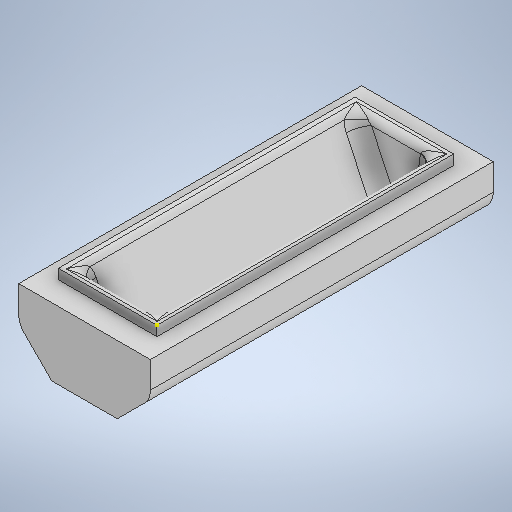
# Autodesk Inventor part: E1-QR-Port
Saved by Autodesk Inventor 2025.2 (Build 292293000, 293)
## iProperties
Created: 2025-11-18
Part Number: E1-QR-Port
Material: 일반
Document SubType Name: Modeling
Designer: RunGeun
Density: 1 g/cm^3
Appearance: 기본값
Author: RunGeun
Autodesk Inventor part; units mm, degrees
ref_plane "YZ Plane" through (0, 0, 0) normal (1, 0, 0) x (0, 1, 0)
ref_plane "XZ Plane" through (0, 0, 0) normal (0, 1, 0) x (-1, 0, 0)
ref_plane "XY Plane" through (0, 0, 0) normal (0, 0, 1) x (1, 0, 0)
sketch "스케치1" plane through (0, 0, 0) normal (0, 1, 0) x (-1, 0, 0)
  line L0 (0, 0) -> (29.8, 0)
  line L1 (29.8, 0) -> (29.8, -89.7)
  line L2 (29.8, -89.7) -> (0, -89.7)
  line L3 (0, -89.7) -> (0, 0)
  line L4 (34.8, 7) -> (-5, 7)
  line L5 (-5, 7) -> (-5, -96.7)
  line L6 (-5, -96.7) -> (34.8, -96.7)
  line L7 (34.8, -96.7) -> (34.8, 7)
  line L8 (16.2, -3) -> (6, -3)
  line L9 (6, -3) -> (6, -86.7)
  line L10 (6, -86.7) -> (16.2, -86.7)
  line L11 (16.2, -86.7) -> (16.2, -3)
  point P0 (11.1, -86.7)
  dimension "d0" = 89.7
  dimension "d1" = 29.8
  dimension "d2" = 7
  dimension "d3" = 5
  dimension "d4" = 7
  dimension "d5" = 5
  dimension "d6" = 3
  dimension "d7" = 3
  dimension "d8" = 13.6
  dimension "d9" = 6
  constraints: 24 end point, 6 parallel, 3 horizontal, 3 perpendicular, 1 midpoint
  measures "d0" distance of L2.end L0.start
  measures "d1" distance of L1.end L2.end
  measures "d2" distance between parallel lines of L6 L2
  measures "d3" distance between parallel lines of L7 L1
  measures "d4" distance between parallel lines of L4 L0
  measures "d5" distance between parallel lines of L5 L3
  measures "d6" distance from line of L2 point (11.1, -86.7)
  measures "d7" distance between parallel lines of L0 L8
  measures "d8" distance between parallel lines of L1 L11
  measures "d9" distance between parallel lines of L3 L9
extrude "돌출1" add sketch "스케치1" along normal blind 20.5 contours L7 L6 L5 L4
extrude "돌출2" add sketch "스케치1" along normal blind 23.5 contours L0 L1 L2 L3
draft "면 구배1" angle 25 pull direction (0, 1, 0) faces at (-16.2, 7.8333, -30.9) fixed edges at (-16.2, 0, -44.85)
draft "면 구배2" angle 8 pull direction (0, 1, 0) faces at (-6, 7.8333, -58.8) fixed edges at (-6, 0, -44.85)
sketch "스케치2" plane through (0, 23.5, 0) normal (0, 1, 0) x (1, 0, 0)
  point P0 (0, 0)
chamfer "모따기1" distance 10 angle 45 2 edges at (-34.8, 0, -44.85) (5, 0, -44.85)
fillet "모깎기1" radius 2 4 edges at (-27.1582, 23.5, -44.85) (-2.6973, 23.5, -44.85) (-14.9278, 23.5, -3) (-14.9278, 23.5, -86.7)
fillet "모깎기2" radius 4 12 edges at (-26.4275, 21.9329, -86.7474) (-27.3578, 23.1868, -87.6254) (-21.2128, 10.75, -86.7) (-2.9588, 21.6395, -86.7049) (-2.2708, 23.0094, -87.3879) (-4.4892, 10.75, -86.7) (-2.9588, 21.6395, -2.9951) (-2.2708, 23.0094, -2.3121) (-4.4892, 10.75, -3) (-26.4275, 21.9329, -2.9526) (-27.3578, 23.1868, -2.0746) (-21.2128, 10.75, -3)
fillet "모깎기3" radius 6 2 edges at (-34.8, 10, -44.85) (5, 10, -44.85)
